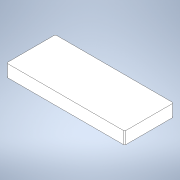
# Autodesk Inventor part: base_of_linear_drive
Saved by Autodesk Inventor 2022 (Build 260153000, 153)
## iProperties
Created: 2022-08-11
Part Number: base_of_linear_drive
Material: Generic
Document SubType Name: Modeling
Designer: Alok
Density: 1 g/cm^3
Appearance: Default
Author: Alok
Autodesk Inventor part; units mm, degrees
ref_plane "YZ Plane" through (0, 0, 0) normal (1, 0, 0) x (0, 1, 0)
ref_plane "XZ Plane" through (0, 0, 0) normal (0, 1, 0) x (-1, 0, 0)
ref_plane "XY Plane" through (0, 0, 0) normal (0, 0, 1) x (1, 0, 0)
sketch "Sketch1" plane through (0, 0, 0) normal (0, 1, 0) x (-1, 0, 0)
  line L0 (145, 60) -> (-145, 60)
  line L1 (-145, 60) -> (-145, -60)
  line L2 (-145, -60) -> (145, -60)
  line L3 (145, -60) -> (145, 60)
  line L4 (145, 60) -> (-145, -60) construction
  line L5 (-145, 60) -> (145, -60) construction
  point P0 (0, 0)
  dimension "d0" = 290
  dimension "d1" = 120
  constraints: 12 end point, 2 midpoint, 2 parallel, 1 horizontal, 1 perpendicular
  measures "d0" distance of L2.end L1.end
  measures "d1" distance of L1.end L0.end
extrude "Extrusion1" add sketch "Sketch1" along normal blind 30
fillet "Face Fillet1" radius 3 1 edges at (-145, 15, -60)
fillet "Face Fillet2" radius 3 1 edges at (-145, 15, 60)
fillet "Face Fillet3" radius 3 1 edges at (145, 15, 60)
fillet "Face Fillet4" radius 3 1 edges at (145, 15, -60)
body "Solid1"
